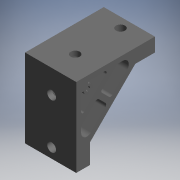
# Autodesk Inventor part: NBLUW8-60_b
Saved by Autodesk Inventor 2017.3 (Build 213256000, 256)
## iProperties
Part Number: NBLUW8-60_b
Material: Generic
Catalog Web Link: www.cadenas.de
Description: NBLUW8-50, HBLUW8-50, HBLUW8-100, NBLUW8-60, HBLUW8-60_body-Brackets for Aluminum Frame 50/60mm Square
Vendor: MISUMI
Document SubType Name: Modeling
Designer: partserver
Manufacturer: MISUMI
Mass: 95.1268 g
Surface Area: 331.48 cm^2
Volume: 95.1268 cm^3
Density: 1 g/cm^3
Appearance: PSOLRGB-128-128-128
Category: PARTsolutions
Company: MISUMI
Title: NBLUW8-60_b
Author: Cadenas PARTsolutions
Comments: Brackets for Aluminum Frame 50/60mm Square
PSOL_IDENT_0: {$CADENAS_DATA\23d-libs\misumi\metric\38_al_extrusions_blackets\8\hbluw8.prj},224 {VTYP=3D},{NB=NBLU
PSOL_IDENT_1: W8-60_b},{LINA=NBLUW8-60_b},{NN=NBLUW8-50, HBLUW8-50, HBLUW8-100, NBLUW8-60, HBLUW8-60_body},{DATE=1
PSOL_IDENT_2: 7.06.2021 07:11:02},{GEOMDATE=14.12.2017 04:33:00},{VERSION=},{LINEID=30},{WBVAR=ALT1,ALT2},{WBNUMER
PSOL_IDENT_3: IC=}  {NB=NBLUW8-60_b},{LINA=NBLUW8-60_b},{KT=DUMMY},{PN=NBLUW8-60},{TS=NBLUW8-60},{MAT=A6063S-T5},{
PSOL_IDENT_4: ST=Clear Anodizing},{MASS=275},{AFS=HFS8-6060},{ALT1=},{ALT1ALG= '', 'w/o C (Mounting Holes for Cove
PSOL_IDENT_5: r)' },{ALT2=},{AB=CBM8-15, CBM8-25},{NOB=2},{AN=HNTT8-8},{NON=4},{M=5},{TAPDEPTH=15},{NO=60},{W=52},
PSOL_IDENT_6: {A1=52.0000},{A2=25.0000},{A3=27.0000},{MAT1=1010 Steel (or Equivalent)},{MAT2=316 Stainless Steel (
PSOL_IDENT_7: or Equivalent)},{TIF=3}
NB: NBLUW8-60_b
NN: NBLUW8-50, HBLUW8-50, HBLUW8-100, NBLUW8-60, HBLUW8-60_body
NT: Brackets for Aluminum Frame 50/60mm Square
NBSYN: $PN._b
LINA: NBLUW8-60_b
CATALOG: Misumi
PN: NBLUW8-60
TS: NBLUW8-60
MAT: A6063S-T5 Aluminum Alloy
ST: Anodize
MASS: 275
AFS: HFS8-6060
ALT1: w/o C (Mounting Holes for Cover)
ALT2: w/o Set of Applicable Bolt and Nut
AB: CBM8-15, CBM8-25
NOB: 2
AN: HNTT8-8
NON: 4
A1: 52
A2: 25
A3: 27
MAT1: 1010 Steel (or Equivalent)
MAT2: 316 Stainless Steel (or Equivalent)
TIF: 3
SUPPLIER: MISUMI
ARTICLENO: NBLUW8-60_b
BOMINFO: NBLUW8-60_b
CREATOR: CADENAS GmbH
Autodesk Inventor part; units mm, degrees
sketch "Sketch_2" plane through (-25, 0, 0) normal (1, 0, 0) x (0, 0, -1)
  line L0 (-80, 0) -> (0, 0)
  line L1 (0, 0) -> (0, 80)
  line L2 (0, 80) -> (-14, 80)
  line L3 (-14, 80) -> (-14, 60.0058)
  line L4 (-14, 60.0058) -> (-60.0058, 14)
  line L5 (-60.0058, 14) -> (-80, 14)
  line L6 (-80, 14) -> (-80, 0)
  arc A0 (-29.5782, 37.3565) -> (-29.5782, 33.1139) centre (-27.4569, 35.2352) ccw
  line L7 (-29.5782, 33.1139) -> (-22.5072, 26.0428)
  arc A1 (-22.5072, 26.0428) -> (-19.6788, 26.0428) centre (-21.093, 27.457) ccw
  line L8 (-19.6788, 26.0428) -> (-5.5858, 40.1357)
  arc A2 (-5.5858, 40.1357) -> (-5, 41.55) centre (-7, 41.55) ccw
  line L9 (-5, 41.55) -> (-5, 47.4494)
  arc A3 (-5, 47.4494) -> (-15.2426, 51.6921) centre (-11, 47.4494) ccw
  line L10 (-15.2426, 51.6921) -> (-29.5782, 37.3565)
  arc A4 (-30.2362, 8.4142) -> (-28.822, 5) centre (-28.822, 7) ccw
  line L11 (-28.822, 5) -> (-13, 5)
  arc A5 (-13, 5) -> (-12, 6) centre (-13, 6) ccw
  line L12 (-12, 6) -> (-12, 7.0251)
  arc A6 (-12, 7.0251) -> (-12.45, 7.5226) centre (-12.5, 7.0251) ccw
  arc A7 (-16.4582, 12.6122) -> (-12.45, 7.5226) centre (-12, 12) ccw
  arc A8 (-15.8334, 13.0271) -> (-16.4582, 12.6122) centre (-15.9628, 12.5442) ccw
  line L13 (-15.8334, 13.0271) -> (-14.4645, 12.6604)
  arc A9 (-14.0951, 12.1433) -> (-14.4645, 12.6604) centre (-14.5939, 12.1774) ccw
  arc A10 (-14.0951, 12.1433) -> (-12.1433, 14.0951) centre (-12, 12) ccw
  arc A11 (-12.6604, 14.4645) -> (-12.1433, 14.0951) centre (-12.1774, 14.5939) ccw
  line L14 (-12.6604, 14.4645) -> (-13.0272, 15.8334)
  arc A12 (-12.6123, 16.4581) -> (-13.0272, 15.8334) centre (-12.5443, 15.9628) ccw
  arc A13 (-7.5226, 12.45) -> (-12.6123, 16.4581) centre (-12, 12) ccw
  arc A14 (-7.5226, 12.45) -> (-7.0251, 12) centre (-7.0251, 12.5) ccw
  line L15 (-7.0251, 12) -> (-6, 12)
  arc A15 (-6, 12) -> (-5, 13) centre (-6, 13) ccw
  line L16 (-5, 13) -> (-5, 28.822)
  arc A16 (-5, 28.822) -> (-8.4142, 30.2362) centre (-7, 28.822) ccw
  line L17 (-8.4142, 30.2362) -> (-30.2362, 8.4142)
  arc A17 (-51.6921, 15.2426) -> (-47.4494, 5) centre (-47.4494, 11) ccw
  line L18 (-47.4494, 5) -> (-41.9642, 5)
  arc A18 (-41.9642, 5) -> (-39.8428, 5.8787) centre (-41.9642, 8) ccw
  line L19 (-39.8428, 5.8787) -> (-26.7498, 18.9717)
  arc A19 (-26.7498, 18.9717) -> (-26.7498, 23.2143) centre (-28.8712, 21.093) ccw
  line L20 (-26.7498, 23.2143) -> (-33.1138, 29.5783)
  arc A20 (-33.1138, 29.5783) -> (-37.3564, 29.5783) centre (-35.2351, 27.457) ccw
  line L21 (-37.3564, 29.5783) -> (-51.6921, 15.2426)
  constraints: 44 end point, 42 point on circle, 21 centre point
extrude "Extrusion1" add sketch "Sketch_2" along normal blind 52
sketch "Sketch_3" plane through (0, 0, 0) normal (1, 0, 0) x (0, 0, -1)
  line L0 (0, 24) -> (-80, 24)
  line L1 (-80, 24) -> (-80, 31)
  line L2 (-80, 31) -> (-5, 31)
  line L3 (-5, 31) -> (-5, 28.5)
  line L4 (-5, 28.5) -> (0, 28.5)
  line L5 (0, 28.5) -> (0, 24)
  line L6 (0, 24) -> (-80, 24)
  constraints: 14 end point
revolve "Revolution1" cut sketch "Sketch_3" angle 360 about axis through (0, 24, 0) along (0, 0, -1)
sketch "Sketch_4" plane through (0, 0, 0) normal (1, 0, 0) x (0, 0, -1)
  line L0 (-24, 80) -> (-24, 0)
  line L1 (-24, 0) -> (-28.5, 0)
  line L2 (-28.5, 0) -> (-28.5, 5)
  line L3 (-28.5, 5) -> (-31, 5)
  line L4 (-31, 5) -> (-31, 80)
  line L5 (-31, 80) -> (-24, 80)
  line L6 (-24, 80) -> (-24, 0)
  constraints: 14 end point
revolve "Revolution2" cut sketch "Sketch_4" angle 360 about axis through (0, 80, 24) along (0, 1, 0)
sketch "Sketch4" plane through (-25, 0, 0) normal (0, 0, -1) x (-1, 0, 0)
  point P0 (-25, 70)
hole "Hole1" at (0, 70, 0) direction (0, 0, 1) diameter 9 depth 15
sketch "Sketch_6" plane through (0, 0, 0) normal (1, 0, 0) x (0, 0, -1)
  line L0 (-70, 15) -> (-70, 0)
  line L1 (-70, 0) -> (-74.5, 0)
  line L2 (-74.5, 0) -> (-74.5, 15)
  line L3 (-74.5, 15) -> (-70, 15)
  line L4 (-70, 15) -> (-70, 0)
  constraints: 10 end point
revolve "Revolution3" cut sketch "Sketch_6" angle 360 about axis through (0, 15, 70) along (0, 1, 0)
ref_plane "bracket_to_dummy_XY" through (0, 0, 0) normal (0, 1, 0) x (1, 0, 0)
ref_plane "bracket_to_dummy_YZ" through (0, 0, 0) normal (1, 0, 0) x (0, 0, -1)
ref_plane "bracket_to_dummy_ZX" through (0, 0, 0) normal (0, 0, -1) x (0, 1, 0)
ref_plane "to_bolt_a_1_XY" through (0, 70, 14) normal (0, 0, 1) x (1, 0, 0)
ref_plane "to_bolt_a_1_YZ" through (0, 70, 14) normal (1, 0, 0) x (0, 1, 0)
ref_plane "to_bolt_a_1_ZX" through (0, 70, 14) normal (0, 1, 0) x (0, 0, 1)
ref_plane "to_bolt_b_1_XY" through (0, 24, 5) normal (0, 0, 1) x (1, 0, 0)
ref_plane "to_bolt_b_1_YZ" through (0, 24, 5) normal (1, 0, 0) x (0, 1, 0)
ref_plane "to_bolt_b_1_ZX" through (0, 24, 5) normal (0, 1, 0) x (0, 0, 1)
ref_plane "to_bolt_base_a_1_XY" through (0, 14, 70) normal (0, 1, 0) x (1, 0, 0)
ref_plane "to_bolt_base_a_1_YZ" through (0, 14, 70) normal (1, 0, 0) x (0, 0, -1)
ref_plane "to_bolt_base_a_1_ZX" through (0, 14, 70) normal (0, 0, -1) x (0, 1, 0)
ref_plane "to_bolt_base_b_1_XY" through (0, 5, 24) normal (0, 1, 0) x (1, 0, 0)
ref_plane "to_bolt_base_b_1_YZ" through (0, 5, 24) normal (1, 0, 0) x (0, 0, -1)
ref_plane "to_bolt_base_b_1_ZX" through (0, 5, 24) normal (0, 0, -1) x (0, 1, 0)
ref_plane "to_nut_a_1_XY" through (0, 70, -6) normal (0, 0, 1) x (1, 0, 0)
ref_plane "to_nut_a_1_YZ" through (0, 70, -6) normal (1, 0, 0) x (0, 1, 0)
ref_plane "to_nut_a_1_ZX" through (0, 70, -6) normal (0, 1, 0) x (0, 0, 1)
ref_plane "to_nut_a_3_XY" through (0, 24, -6) normal (0, 0, 1) x (1, 0, 0)
ref_plane "to_nut_a_3_YZ" through (0, 24, -6) normal (1, 0, 0) x (0, 1, 0)
ref_plane "to_nut_a_3_ZX" through (0, 24, -6) normal (0, 1, 0) x (0, 0, 1)
ref_plane "to_nut_base_a_1_XY" through (0, -6, 70) normal (0, 1, 0) x (1, 0, 0)
ref_plane "to_nut_base_a_1_YZ" through (0, -6, 70) normal (1, 0, 0) x (0, 0, -1)
ref_plane "to_nut_base_a_1_ZX" through (0, -6, 70) normal (0, 0, -1) x (0, 1, 0)
ref_plane "to_nut_base_a_3_XY" through (0, -6, 24) normal (0, 1, 0) x (1, 0, 0)
ref_plane "to_nut_base_a_3_YZ" through (0, -6, 24) normal (1, 0, 0) x (0, 0, -1)
ref_plane "to_nut_base_a_3_ZX" through (0, -6, 24) normal (0, 0, -1) x (0, 1, 0)
body "Solid1"
